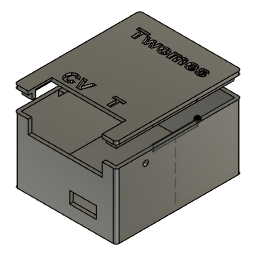
OpenThermEnclosure (Autodesk Fusion 360 design; units mm, degrees)
Autodesk Fusion 360 part; units mm, degrees
sketch "Sketch1" plane through (0, 0, 0) normal (0, 0, 1) x (1, 0, 0)
  line L0 (0, 0) -> (34.4, 0)
  line L1 (34.4, 0) -> (34.4, -42.4)
  line L2 (34.4, -42.4) -> (0, -42.4)
  line L3 (0, -42.4) -> (0, 0)
  dimension "d6" = 34.4
  dimension "d7" = 42.4
  constraint horizontal L0
  constraint vertical L1
  constraint horizontal L2
  constraint vertical L3
  constraint coincident L0.start L3.end
  measures "d6" distance of L0.start L0.end
  measures "d7" distance of L0.start L2.end
extrude "Extrude1" add sketch "Sketch1" along normal blind 22 makes body 1
shell "Shell1" thickness 1.2 removed faces 1 at (11.4667, -28.2667, 22) on bodies 1
sketch "Sketch2" plane through (0, -42.4, 0) normal (0, -1, 0) x (1, 0, 0)
  line L0 (0, 0) -> (34.4, 0)
  line L1 (34.4, 0) -> (34.4, 22)
  line L2 (34.4, 22) -> (0, 22)
  line L3 (0, 22) -> (0, 0)
  line L4 (4.7, 22) -> (29.7, 22)
  line L5 (29.7, 22) -> (29.7, 20)
  line L6 (29.7, 20) -> (4.7, 20)
  line L7 (4.7, 20) -> (4.7, 22)
  dimension "d11" = 25
  dimension "d12" = 2
  constraint horizontal L4
  constraint vertical L5
  constraint horizontal L6
  constraint vertical L7
  constraint collinear L2 L4
  measures "d11" distance of L4.start L4.end
  measures "d12" distance of L4.start L6.end
extrude "Extrude2" cut sketch "Sketch2" against normal blind 2 contours L2 L4 L5 L6 L7 bodies 1
sketch "Sketch3" plane through (0, -41.2, 0) normal (0, 1, 0) x (-1, 0, 0)
  line L0 (-4.7, 22) -> (-4.7, 20)
  line L1 (-4.7, 20) -> (-29.7, 20)
  line L2 (-29.7, 20) -> (-29.7, 22)
  line L3 (-29.7, 22) -> (-33.2, 22)
  line L4 (-33.2, 22) -> (-33.2, 1.2)
  line L5 (-33.2, 1.2) -> (-1.2, 1.2)
  line L6 (-1.2, 1.2) -> (-1.2, 22)
  line L7 (-1.2, 22) -> (-4.7, 22)
  line L8 (-27.7, 8.2) -> (-18.7, 8.2)
  line L9 (-18.7, 8.2) -> (-18.7, 4.2)
  line L10 (-18.7, 4.2) -> (-27.7, 4.2)
  line L11 (-27.7, 4.2) -> (-27.7, 8.2)
  dimension "d17" = 9
  dimension "d18" = 4
  dimension "d19" = 5.5
  dimension "d20" = 3
  constraint horizontal L8
  constraint vertical L9
  constraint horizontal L10
  constraint vertical L11
  measures "d17" distance of L8.start L8.end
  measures "d18" distance of L8.start L10.end
  measures "d19" distance of L4 L11
  measures "d20" distance of L5 L10
extrude "Extrude3" cut sketch "Sketch3" against normal blind 3 contours L8 L9 L10 L11 bodies 1
sketch "Sketch1 (2)" plane through (0, 0, 22) normal (0, 0, 1) x (-1, 0, 0) in component "top"
  line L0 (-4.7, 42.4) -> (-4.7, 41.2)
  line L1 (-4.7, 41.2) -> (-1.2, 41.2)
  line L2 (-1.2, 41.2) -> (-1.2, 1.2)
  line L3 (-1.2, 1.2) -> (-33.2, 1.2)
  line L4 (-33.2, 1.2) -> (-33.2, 41.2)
  line L5 (-33.2, 41.2) -> (-29.7, 41.2)
  line L6 (-29.7, 41.2) -> (-29.7, 42.4)
  line L7 (-29.7, 42.4) -> (-34.4, 42.4)
  line L8 (-34.4, 42.4) -> (-34.4, 0)
  line L9 (-34.4, 0) -> (0, 0)
  line L10 (0, 0) -> (0, 42.4)
  line L11 (0, 42.4) -> (-4.7, 42.4)
  line L12 (0, 0) -> (-34.4, 0)
  line L13 (-34.4, 0) -> (-34.4, 42.4)
  line L14 (-34.4, 42.4) -> (0, 42.4)
  line L15 (0, 42.4) -> (0, 0)
  line L16 (-29.7, 42.4) -> (-6.2653, 42.4)
  line L17 (-6.2653, 42.4) -> (-6.2653, 38.4)
  line L18 (-6.2653, 38.4) -> (-29.7, 38.4)
  line L19 (-29.7, 38.4) -> (-29.7, 42.4)
  dimension "d23" = 34.4
  dimension "d24" = 42.4
  dimension "d25" = 23.4347
  dimension "d26" = 4
  constraint horizontal L12
  constraint vertical L13
  constraint horizontal L14
  constraint vertical L15
  constraint coincident L9.end L10.start
  constraint horizontal L16
  constraint vertical L17
  constraint horizontal L18
  constraint vertical L19
  constraint coincident L6.end L7.start
  measures "d23" distance of L9.end L8.end
  measures "d24" distance of L9.end L10.end
  measures "d25" distance of L6.end L16.end
  measures "d26" distance of L6.end L18.end
extrude "Extrude1'" add sketch "Sketch1 (2)" along normal blind 1.2 separate body contours L0 L1 L2 L3 L4 L5 L6 L7 L8 L9 L10 L11 L12 L13 L14 L15 L19 | L0 L1 L2 L3 L4 L5 L14 L17 L18 L19 makes body 2 in component "top"
sketch "Sketch2 (2)" plane through (0, 0, 22) normal (0, 0, -1) x (1, 0, 0) in component "top"
  line L0 (6.2653, 38.4) -> (6.2653, 42.4)
  line L1 (6.2653, 42.4) -> (0, 42.4)
  line L2 (0, 42.4) -> (0, 0)
  line L3 (0, 0) -> (34.4, 0)
  line L4 (34.4, 0) -> (34.4, 42.4)
  line L5 (34.4, 42.4) -> (29.7, 42.4)
  line L6 (29.7, 42.4) -> (29.7, 38.4)
  line L7 (29.7, 38.4) -> (6.2653, 38.4)
  line L8 (33.1, 1.3) -> (1.3, 1.3)
  line L9 (1.3, 1.3) -> (1.3, 41.1)
  line L10 (1.3, 41.1) -> (33.1, 41.1)
  line L11 (33.1, 41.1) -> (33.1, 1.3)
  dimension "d29" = 31.8
  dimension "d30" = 39.8
  dimension "d31" = 1.3
  dimension "d32" = 1.3
  dimension "d33" = 1.3
  dimension "d34" = 1.3
  constraint horizontal L8
  constraint vertical L9
  constraint horizontal L10
  constraint vertical L11
  measures "d29" distance of L8.start L8.end
  measures "d30" distance of L8.start L10.end
  measures "d31" distance of L4 L11
  measures "d32" distance of L2 L9
  measures "d33" distance of L3 L8
  measures "d34" distance of L1 L10
extrude "Extrude2'" add sketch "Sketch2 (2)" along normal blind 2 contours L0 L6 L7 L8 L9 L10 L11 bodies 2 in component "top"
shell "Shell1'" thickness 1.2 removed faces 1 at (13.5551, -13.6667, 20) on bodies 2 in component "top"
sketch "Sketch3 (2)" plane through (-0.2008, 0.1083, 20) normal (0, 0, -1) x (1, 0, 0) in component "top"
  line L0 (31.1008, 40.0083) -> (32.1008, 40.0083)
  line L1 (32.1008, 40.0083) -> (32.1008, 2.6083)
  line L2 (32.1008, 2.6083) -> (2.7008, 2.6083)
  line L3 (2.7008, 2.6083) -> (2.7008, 40.0083)
  line L4 (2.7008, 40.0083) -> (5.2661, 40.0083)
  line L5 (5.2661, 40.0083) -> (5.2661, 37.3083)
  line L6 (5.2661, 37.3083) -> (31.1008, 37.3083)
  line L7 (31.1008, 37.3083) -> (31.1008, 40.0083)
  line L8 (29.9008, 41.2083) -> (29.9008, 38.5083)
  line L9 (29.9008, 38.5083) -> (6.4661, 38.5083)
  line L10 (6.4661, 38.5083) -> (6.4661, 41.2083)
  line L11 (6.4661, 41.2083) -> (1.5008, 41.2083)
  line L12 (1.5008, 41.2083) -> (1.5008, 1.4083)
  line L13 (1.5008, 1.4083) -> (33.3008, 1.4083)
  line L14 (33.3008, 1.4083) -> (33.3008, 41.2083)
  line L15 (33.3008, 41.2083) -> (29.9008, 41.2083)
  line L16 (5.2661, 40.0083) -> (6.4661, 40.0083)
  line L17 (31.1008, 40.0083) -> (29.9008, 40.0083)
  constraint coincident L4.end L5.start
  constraint coincident L10 L16.end
  constraint perpendicular L10 L16
  constraint coincident L0.start L7.end
  constraint coincident L8 L17.end
  constraint perpendicular L8 L17
extrude "Extrude3'" cut sketch "Sketch3 (2)" against normal blind 2 contours L5 L6 L7 L8 L9 L10 L16 L17 bodies 2 in component "top"
sketch "Sketch4" plane through (33.2, 0, 0) normal (-1, 0, 0) x (0, -1, 0)
  line L0 (1.2, 1.2) -> (41.2, 1.2)
  line L1 (41.2, 1.2) -> (41.2, 22)
  line L2 (41.2, 22) -> (1.2, 22)
  line L3 (1.2, 22) -> (1.2, 1.2)
  line L4 (13.7, 22) -> (28.7, 22)
  line L5 (28.7, 22) -> (28.7, 20)
  line L6 (28.7, 20) -> (13.7, 20)
  line L7 (13.7, 20) -> (13.7, 22)
  line L8 (21.2, 1.2) -> (21.2, 20) construction
  dimension "d40" = 15
  dimension "d41" = 2
  constraint horizontal L4
  constraint vertical L5
  constraint horizontal L6
  constraint vertical L7
  constraint coincident L2 L4.start
  constraint midpoint L0 L8.start
  constraint midpoint L6 L8.end
  constraint perpendicular L6 L8
  measures "d40" distance of L4.start L4.end
  measures "d41" distance of L4.start L6.end
extrude "Extrude4" add sketch "Sketch4" along normal blind 5 draft -45 contours L2 L4 L5 L6 L7 bodies 1
ref_plane "WorkPlane1" through (17.2, -21.2, 11.6) normal (-1, 0, 0) x (0, -1, 0)
mirror "Mirror1" about plane through (17.2, -21.2, 11.6) normal (-1, 0, 0) of "Extrude4"
extrude "Extrude4'" cut sketch "Sketch4" along normal blind 5 draft -45 from surface at 0.1 contours L2 L4 L5 L6 L7 bodies 2 in component "top"
mirror "Mirror1'" about plane through (17.2, -21.2, 11.6) normal (-1, 0, 0) of "Extrude4'" in component "top"
sketch "Sketch4 (2)" plane through (0, 0, 22) normal (0, 0, -1) x (1, 0, 0) in component "top"
  line L0 (6.2653, 39.9) -> (2.5, 39.9)
  line L1 (2.5, 39.9) -> (2.5, 2.5)
  line L2 (2.5, 2.5) -> (31.9, 2.5)
  line L3 (31.9, 2.5) -> (31.9, 39.9)
  line L4 (31.9, 39.9) -> (29.7, 39.9)
  line L5 (29.7, 39.9) -> (29.7, 38.4)
  line L6 (29.7, 38.4) -> (6.2653, 38.4)
  line L7 (6.2653, 38.4) -> (6.2653, 39.9)
  line L8 (29.7, 38.4) -> (31.9, 38.4)
  line L9 (31.9, 38.4) -> (31.9, 39.9)
  line L10 (31.9, 39.9) -> (29.7, 39.9)
  line L11 (29.7, 39.9) -> (29.7, 38.4)
  line L12 (6.2653, 38.4) -> (2.5, 38.4)
  line L13 (2.5, 38.4) -> (2.5, 39.9)
  line L14 (2.5, 39.9) -> (6.2653, 39.9)
  line L15 (6.2653, 39.9) -> (6.2653, 38.4)
  constraint horizontal L8
  constraint vertical L9
  constraint horizontal L10
  constraint vertical L11
  constraint coincident L3.end L4.start
  constraint coincident L5.end L6.start
  constraint horizontal L12
  constraint vertical L13
  constraint horizontal L14
  constraint vertical L15
  constraint coincident L0.end L1.start
  constraint coincident L6.end L7.start
extrude "Extrude5" cut sketch "Sketch4 (2)" against normal blind 0.5 contours L0 L1 L7 L12 L13 L14 L15 | L3 L4 L5 L8 L9 L10 L11 bodies 2 in component "top"
extrude "Extrude6" cut 1 faces at (6.2653, -40.3, 21.5) along direction (-1, 0, 0) blind 1.6 on bodies 2 bodies 2 in component "top"
sketch "Sketch5" plane through (34.4, 0, 0) normal (1, 0, 0) x (0, 1, 0) in component "top"
  line L0 (-42.4, 0) -> (0, 0)
  line L1 (0, 0) -> (0, 22)
  line L2 (0, 22) -> (-42.4, 22)
  line L3 (-42.4, 22) -> (-42.4, 0)
  circle A0 centre (-32.4, 19) radius 0.9
  dimension "d55" = 1.8
  dimension "d65" = 10
  dimension "d74" = 3
  measures "d55" diameter of A0
  measures "d65" distance of L3 A0.centre
  measures "d74" distance of L2 A0.centre
extrude "Extrude5'" cut sketch "Sketch5" against normal blind 2 contours A0 bodies 1
extrude "Extrude7" cut sketch "Sketch5" against normal blind 2 contours A0 bodies 2 in component "top"
sketch "Sketch5 (2)" plane through (1.2, 0, 0) normal (1, 0, 0) x (0, 1, 0)
  line L0 (-28.7, 20) -> (-28.7, 22)
  line L1 (-28.7, 22) -> (-41.2, 22)
  line L2 (-41.2, 22) -> (-41.2, 1.2)
  line L3 (-41.2, 1.2) -> (-1.2, 1.2)
  line L4 (-1.2, 1.2) -> (-1.2, 22)
  line L5 (-1.2, 22) -> (-13.7, 22)
  line L6 (-13.7, 22) -> (-13.7, 20)
  line L7 (-13.7, 20) -> (-28.7, 20)
  circle A0 centre (-37, 6.9) radius 1
  dimension "d60" = 2
  dimension "d66" = 4.2
  dimension "d69" = 5.7
  measures "d60" diameter of A0
  measures "d66" distance of L2 A0.centre
  measures "d69" distance of L3 A0.centre
extrude "Extrude8" cut 1 faces at (13.0102, -38.4, 22.9667) along direction (0, 1, 0) blind 4 on bodies 2 bodies 2 in component "top"
extrude "Extrude7'" cut 1 faces at (21.3667, -42, 20) along direction (0, 0, -1) blind 2.5 on bodies 1 bodies 1
sketch "Sketch6" plane through (0, 0, 1.2) normal (0, 0, 1) x (-1, 0, 0)
  line L0 (-1.2, 41.2) -> (-33.2, 41.2)
  line L1 (-33.2, 41.2) -> (-33.2, 1.2)
  line L2 (-33.2, 1.2) -> (-1.2, 1.2)
  line L3 (-1.2, 1.2) -> (-1.2, 41.2)
  line L4 (-29, 40) -> (-26.5, 40)
  line L5 (-26.5, 40) -> (-26.5, 37.5)
  line L6 (-26.5, 37.5) -> (-29, 37.5)
  line L7 (-29, 37.5) -> (-29, 40)
  dimension "d70" = 2.5
  dimension "d71" = 2.5
  constraint horizontal L4
  constraint vertical L5
  constraint horizontal L6
  constraint vertical L7
  measures "d70" distance of L4.start L4.end
  measures "d71" distance of L4.start L6.end
extrude "Extrude8'" add sketch "Sketch6" along normal blind 2.5 contours L4 L5 L6 L7 bodies 1
fillet "Fillet1" radius 1 4 edges at (34.4, 0, 11) (0, 0, 11) (0, -42.4, 11) (34.4, -42.4, 11) on bodies 1
fillet "Fillet1'" radius 1 4 edges at (34.4, 0, 22.6) (0, 0, 22.6) (0, -42.4, 22.6) (34.4, -42.4, 22.6) on bodies 2 in component "top"
move_body "Move1" bodies 2 to x (1, 0, 0) y (0, 1, 0) z (0, 0, 1) at (0, 0, 7) in component "top"
sketch "Sketch7" plane through (0, 0, 30.2) normal (0, 0, 1) x (-1, 0, 0)
  arc A0 (-33.4, 42.4) -> (-34.4, 41.4) centre (-33.4, 41.4) ccw
  line L0 (-34.4, 41.4) -> (-34.4, 1)
  arc A1 (-34.4, 1) -> (-33.4, 0) centre (-33.4, 1) ccw
  line L1 (-33.4, 0) -> (-1, 0)
  arc A2 (-1, 0) -> (0, 1) centre (-1, 1) ccw
  line L2 (0, 1) -> (0, 41.4)
  arc A3 (0, 41.4) -> (-1, 42.4) centre (-1, 41.4) ccw
  line L3 (-1, 42.4) -> (-4.6653, 42.4)
  line L4 (-4.6653, 42.4) -> (-4.6653, 34.4)
  line L5 (-4.6653, 34.4) -> (-29.7, 34.4)
  line L6 (-29.7, 34.4) -> (-29.7, 42.4)
  line L7 (-29.7, 42.4) -> (-33.4, 42.4)
  line L8 (-6.0431, 33.1651) -> (-13.0431, 33.1651) construction
  line L9 (-13.0431, 33.1651) -> (-13.0431, 29.1651) construction
  line L10 (-13.0431, 29.1651) -> (-6.0431, 29.1651) construction
  line L11 (-6.0431, 29.1651) -> (-6.0431, 33.1651) construction
  line L12 (-20.7548, 32.7792) -> (-24.7361, 32.7876) construction
  line L13 (-24.7361, 32.7876) -> (-24.7439, 29.0773) construction
  line L14 (-24.7439, 29.0773) -> (-20.7625, 29.0689) construction
  line L15 (-20.7625, 29.0689) -> (-20.7548, 32.7792) construction
  line L16 (-5, 10) -> (-30, 10) construction
  line L17 (-30, 10) -> (-30, 5) construction
  line L18 (-30, 5) -> (-5, 5) construction
  line L19 (-5, 5) -> (-5, 10) construction
  dimension "d79" = 4
  dimension "d80" = 4
  dimension "d83" = 4
  text T0 "CV" font "Arial Black" height 4 align left top in box 7 x 4 at (-6.0431, 33.1651) x (-1, 0) y (0, -1) spacing 1 kerned
  text T1 "T" font "Arial Black" height 4 align left top in box 3.9814 x 3.7103 at (-20.7548, 32.7792) x (-0.999998, 0.002093) y (-0.002093, -0.999998) spacing 1 kerned
  text T2 "Twomes" font "Arial Black" height 4 align centre top in box 25 x 5 at (-5, 10) x (-1, 0) y (0, -1) spacing 1 kerned
extrude "Extrude10" cut sketch "Sketch7" against normal blind 0.8 text T2 bodies 2 in component "top"
extrude "Extrude9" cut sketch "Sketch7" against normal blind 0.8 text T1 T0 bodies 2 in component "top"
component "top" placed x (1, 0, 0) y (0, 1, 0) z (0, 0, 1) at (0, 0, 0)
component "Box" placed x (1, 0, 0) y (0, 1, 0) z (0, 0, 1) at (0, 0, 0) in component "top"
equation "Width = 32 mm"
equation "Length = 40 mm"
equation "Height = 22 mm"
equation "screwConnWidth = 25 mm"
equation "Shell = 1.2 mm"
equation "d6 = 2 * Shell + Width"
equation "d7 = 2 * Shell + Length"
equation "d8 = Height"
equation "d10 = Shell"
equation "d11 = screwConnWidth"
equation "USBWIdth = 9 mm"
equation "USBHeight = 4 mm"
equation "d17 = USBWIdth"
equation "d18 = USBHeight"
equation "d23 = 2 * Shell + Width"
equation "d24 = 2 * Shell + Length"
equation "d27 = Shell"
equation "d29 = Width - 0.2 mm"
equation "d30 = Length - 0.2 mm"
equation "d31 = Shell + 0.1 mm"
equation "d33 = Shell + 0.1 mm"
equation "d37 = Shell"
